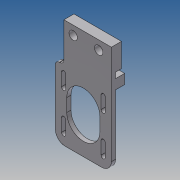
# Autodesk Inventor part: J008087
Saved by Autodesk Inventor 2018.3 (Build 223284000, 284)
## iProperties
Created: 2019-09-05
Material: ALUMINUM, 6061-T651
Vendor: HHMI: JRC - ID&F
Document SubType Name: Modeling
Designer: arnoldj
Density: 2.7 g/cm^3
Appearance: Metal-AL-6061 (Machined)
Part Number: J008087
Project: COMMON
Description: BBP GONIO MOTOR SHIFT PLATE
RuleStatus: InUse
AfterDocSave0: file://Part Number Cleaner
LAB/DEPT: COMMON
REQUESTING SCIENTIST: PACHITARIU, MARIUS
SURFACE ROUGHNESS: 63 Ra
DESIGN DEPARTMENT: HHMI: JRC - ID&F
SPECIAL FINISH: ANODIZE PER MIL-A-8625F, TYPE II, CLASS 2 (BLACK)
ALTERED ITEM PART NUMBER: N/A
ALTERED ITEM VENDOR: N/A
ALTERED ITEM DESCRIPTION: N/A
Author: arnoldj
Revision Number: -
Autodesk Inventor part; units mm, degrees
note: some values were not read from the file. Chosen so that the rebuilt part matches the saved one: edges of "Fillet3".
ref_plane "YZ Plane" through (0, 0, 0) normal (1, 0, 0) x (0, 1, 0)
ref_plane "XZ Plane" through (0, 0, 0) normal (0, 1, 0) x (-1, 0, 0)
sketch "Sketch1" plane through (0, 0, 0) normal (0, 0, 1) x (1, 0, 0)
  line L0 (0, 128.9005) -> (0, -151.1555) projected
  line L1 (-57.1993, 0) -> (35.1957, 0) projected
  line L2 (21.9964, -103.8925) -> (-21.9964, -103.8925)
  line L3 (-21.9964, -103.8925) -> (-21.9964, -18.4723)
  line L4 (-21.9964, -18.4723) -> (21.9964, -18.4723)
  line L5 (21.9964, -18.4723) -> (21.9964, -103.8925)
  line L6 (21.9964, -103.8925) -> (-21.9964, -18.4723) construction
  line L7 (-21.9964, -103.8925) -> (21.9964, -18.4723) construction
  line L8 (15.5, -90.8175) -> (-15.5, -90.8175) construction
  line L9 (-15.5, -90.8175) -> (-15.5, -59.8175) construction
  line L10 (-15.5, -59.8175) -> (15.5, -59.8175) construction
  line L11 (15.5, -59.8175) -> (15.5, -90.8175) construction
  line L12 (15.5, -90.8175) -> (-15.5, -59.8175) construction
  line L13 (-15.5, -90.8175) -> (15.5, -59.8175) construction
  line L14 (0, -111.1475) -> (0, -39.4875) construction
  line L15 (-15.5, -64.8975) -> (-15.5, -54.7375) construction
  line L16 (-13.849, -64.8975) -> (-13.849, -54.7375)
  line L17 (-17.151, -54.7375) -> (-17.151, -64.8975)
  arc A0 (-17.151, -64.8975) -> (-13.849, -64.8975) centre (-15.5, -64.8975) ccw
  arc A1 (-13.849, -54.7375) -> (-17.151, -54.7375) centre (-15.5, -54.7375) ccw
  arc A2 (17.151, -54.7375) -> (13.849, -54.7375) centre (15.5, -54.7375) ccw
  line L18 (17.151, -64.8975) -> (17.151, -54.7375)
  line L19 (15.5, -64.8975) -> (15.5, -54.7375) construction
  line L20 (13.849, -54.7375) -> (13.849, -64.8975)
  arc A3 (13.849, -64.8975) -> (17.151, -64.8975) centre (15.5, -64.8975) ccw
  arc A4 (-13.849, -85.7375) -> (-17.151, -85.7375) centre (-15.5, -85.7375) ccw
  line L21 (-13.849, -95.8975) -> (-13.849, -85.7375)
  line L22 (-15.5, -95.8975) -> (-15.5, -85.7375) construction
  line L23 (-17.151, -85.7375) -> (-17.151, -95.8975)
  arc A5 (-17.151, -95.8975) -> (-13.849, -95.8975) centre (-15.5, -95.8975) ccw
  arc A6 (17.151, -85.7375) -> (13.849, -85.7375) centre (15.5, -85.7375) ccw
  line L24 (17.151, -95.8975) -> (17.151, -85.7375)
  line L25 (15.5, -95.8975) -> (15.5, -85.7375) construction
  line L26 (13.849, -85.7375) -> (13.849, -95.8975)
  arc A7 (13.849, -95.8975) -> (17.151, -95.8975) centre (15.5, -95.8975) ccw
  line L27 (0, -70.2375) -> (0, -80.3975) construction
  line L28 (13.0175, -70.2375) -> (13.0175, -80.3975)
  line L29 (-13.0175, -80.3975) -> (-13.0175, -70.2375)
  arc A8 (13.0175, -70.2375) -> (-13.0175, -70.2375) centre (0, -70.2375) ccw
  arc A9 (-13.0175, -80.3975) -> (13.0175, -80.3975) centre (0, -80.3975) ccw
  point P0 (0, -75.3175)
  point P1 (-44, 88.8925)
  point P2 (15.5, -59.8175)
  point P3 (-15.5, -90.8175)
  point P4 (15.5, -90.8175)
  point P5 (0, -75.3175)
  dimension "d5" = 31
  dimension "d6" = 31
  dimension "d10" = 28.575
  dimension "d11" = 3.302
  dimension "d12" = 10.16
  dimension "d15" = 31
  dimension "d18" = 31
  dimension "d45" = 5.08
  dimension "d51" = 43.9928
  dimension "d62" = 5.08
  dimension "d63" = 85.4202
  dimension "d77" = 21.9964
  constraints: 68 end point, 20 point on circle, 10 centre point, 8 tangent, 6 parallel, 4 midpoint, 4 point on line, 3 horizontal, 2 perpendicular, 2 vertical, 1 coincident, 36 other
  measures "d5" distance of L10.end L8.start
  measures "d6" distance of L9.end L10.end
  measures "d10" distance from line of point (0, -75.318) L2
  measures "d11" distance between parallel lines of L16 L17
  measures "d12" distance of L17.start L17.end
  measures "d15" distance of L15.end L19.end
  measures "d18" distance of L15.end L22.end
  measures "d45" distance of L27.end point (0, -75.318)
  measures "d51" distance of L3.end L4.end
  measures "d62" distance of point (0, -75.318) L27.start
  measures "d63" distance of L2.end L3.end
  measures "d77" distance between parallel lines of L0 L5
extrude "Extrusion1" add sketch "Sketch1" along normal blind 3.302
extrude "Extrusion3" cut sketch "Sketch1" along normal through all contours A8 L28 A9 L0 | L0 A9 L29 A8
sketch "Sketch3" plane through (0, 0, 3.302) normal (0, 0, 1) x (1, 0, 0)
  point P0 (0, 0)
  point P1 (-44, 68.8925)
  point P2 (44, 88.8925)
  point P3 (44, 68.8925)
  point P4 (-44, 88.8925)
hole "Hole2" at (-44, 68.8925, 3.302) at (44, 88.8925, 3.302) at (44, 68.8925, 3.302) at (-44, 88.8925, 3.302) direction (0, 0, -1) diameter 7.0104 end through all clearance for "Socket Head Cap Screw" size "M6" standard "Ansi Metric M Profile"
sketch "Sketch5" plane through (0, 0, 0) normal (1, 0, 0) x (0, 1, 0)
  line L0 (-18.4723, 0) -> (-103.8925, 0) projected
  line L1 (-18.4723, 0) -> (-18.4723, 3.302) projected
  line L2 (-103.8925, 3.302) -> (-18.4723, 3.302) projected
  line L3 (-103.8925, 0) -> (-103.8925, 3.302) projected
  line L4 (-18.4723, 0) -> (-103.8925, 0) projected
  line L5 (-18.4723, 0) -> (-49.1047, 0)
  line L6 (-49.1047, 0) -> (-49.1047, -4.572)
  line L7 (-49.1047, -4.572) -> (-18.4723, -4.572)
  line L8 (-18.4723, -4.572) -> (-18.4723, 0)
  line L9 (-49.1047, -4.572) -> (-41.4847, -4.572)
  line L10 (-41.4847, -4.572) -> (-41.4847, -7.112)
  line L11 (-41.4847, -7.112) -> (-49.1047, -7.112)
  line L12 (-49.1047, -7.112) -> (-49.1047, -4.572)
  point P0 (0, 0)
  dimension "d70" = 23.0124
  dimension "d71" = 7.62
  dimension "d72" = 4.572
  dimension "d73" = 2.54
  constraints: 16 end point, 4 parallel, 2 horizontal, 2 perpendicular
  measures "d70" distance between parallel lines of L8 L10
  measures "d71" distance of L10.end L11.end
  measures "d72" distance between parallel lines of L0 L7
  measures "d73" distance between parallel lines of L7 L11
extrude "Extrusion4" add sketch "Sketch5" against normal blind 15.24 and the other way blind 21.9964 contours L8 L7 L6 L0 | L7 L10 L11 L12
fillet "Fillet2" radius 7.62 2 edges at (-21.9964, -103.8925, 1.651) (21.9964, -103.8925, 1.651)
sketch "Sketch6" plane through (0, 0, 3.302) normal (0, 0, 1) x (1, 0, 0)
  line L0 (-15.24, -41.4847) -> (21.9964, -41.4847) projected
  line L1 (21.9964, -96.2725) -> (21.9964, -18.4723) projected
  point P0 (0, 0)
  point P1 (11.9964, -25.4827)
  point P2 (-8.0036, -25.4827)
  dimension "d78" = 10
  dimension "d79" = 20
  dimension "d80" = 16.002
  constraints: 1 horizontal alignment
  measures "d78" distance from line of point (11.996, -25.483) L1
  measures "d79" distance of point (-8.004, -25.483) point (11.996, -25.483)
  measures "d80" distance from line of point (-8.004, -25.483) L0
hole "Hole4" at (-8.0036, -25.4827, 3.302) at (11.9964, -25.4827, 3.302) direction (0, 0, -1) diameter 6.604 end through all clearance for "Socket Head Cap Screw" size "M6" standard "Ansi Metric M Profile"
sketch "Sketch7" plane through (0, 0, 0) normal (0, 0, -1) x (-1, 0, 0)
  line L0 (15.24, -41.4847) -> (15.24, -49.1047) projected
  line L1 (15.24, -49.1047) -> (-21.9964, -49.1047) projected
  line L2 (21.9964, -18.4723) -> (15.24, -18.4723) projected
  line L3 (21.9964, -96.2725) -> (21.9964, -18.4723) projected
  line L4 (15.24, -49.1047) -> (21.9964, -49.1047)
  line L5 (21.9964, -49.1047) -> (21.9964, -18.4723)
  line L6 (21.9964, -18.4723) -> (15.24, -18.4723)
  line L7 (15.24, -18.4723) -> (15.24, -49.1047)
  point P0 (0, 0)
  constraints: 8 end point, 2 parallel, 1 horizontal, 1 perpendicular
extrude "Extrusion5" cut sketch "Sketch7" against normal up to next
fillet "Fillet3" radius 3.175 2 edges at (-15.24, -49.1047, 1.651) (-21.9964, -49.1047, 1.651)
sketch "Sketch8" plane through (21.9964, -41.4847, -4.572) normal (0, 0, -1) x (-1, 0, 0)
  circle A0 centre (30, 16.002) radius 3.302 projected
  circle A1 centre (10, 16.002) radius 3.302 projected
  line L0 (37.2364, 0) -> (0, 0) projected
  line L1 (37.2364, 23.0124) -> (37.2364, 0) projected
  line L2 (37.2364, 23.0124) -> (0, 23.0124) projected
  line L3 (0, 0) -> (0, 23.0124) projected
  line L4 (0, 0) -> (8.89, 0)
  line L5 (8.89, 0) -> (8.89, 4.445)
  line L6 (8.89, 4.445) -> (0, 4.445)
  line L7 (0, 4.445) -> (0, 0)
  point P0 (21.9964, 41.4847)
  dimension "d91" = 4.445
  dimension "d92" = 8.89
  constraints: 8 end point, 2 parallel, 1 horizontal, 1 perpendicular
  measures "d91" distance of L4.end L5.end
  measures "d92" distance of L5.end L6.end
extrude "Extrusion6" cut sketch "Sketch8" against normal up to surface (4.572 mm away) contours L0 L3 L6 L5
fillet "Fillet4" radius 2.032 2 edges at (13.1064, -41.4847, -2.286) (13.1064, -37.0397, -2.286)
equation "\"d15\" = d6"
equation "\"d18\" = d6"
equation "\"d77\" = 0.5 * d51"
equation "\"d74\" = 0.5 * d51"
body "Solid1"
